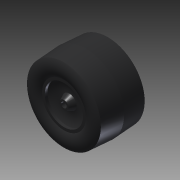
# Autodesk Inventor part: launcher_wheel
Saved by Autodesk Inventor 2013 (Build 170138000, 138)
## iProperties
Created: 2013-07-24
Part Number: launcher_wheel
Material: Generic
Document SubType Name: Modeling
Designer: dkboone
Density: 1 g/cm^3
Author: dkboone
Autodesk Inventor part; units mm, degrees
ref_plane "YZ Plane" through (0, 0, 0) normal (1, 0, 0) x (0, 1, 0)
ref_plane "XZ Plane" through (0, 0, 0) normal (0, 1, 0) x (-1, 0, 0)
ref_plane "XY Plane" through (0, 0, 0) normal (0, 0, 1) x (1, 0, 0)
sketch "Sketch1" plane through (0, 0, 0) normal (1, 0, 0) x (0, 1, 0)
  line L0 (1.5875, -19.05) -> (1.5875, 12.7)
  line L1 (1.5875, 12.7) -> (2.5875, 12.7)
  line L2 (2.5875, 12.7) -> (4.175, 9.525)
  arc A0 (4.175, 9.525) -> (11.1125, 11.1125) centre (5.6612, 18.9827) ccw
  line L3 (11.1125, 11.1125) -> (11.1125, 12.7)
  line L4 (11.1125, 12.7) -> (12.7, 12.7)
  line L5 (21.4312, 12.7) -> (22.225, 0)
  line L6 (18.2563, -12.7) -> (18.2562, 6.35)
  line L7 (18.2562, 6.35) -> (3.9688, 6.35)
  line L8 (3.9688, 6.35) -> (3.9688, -19.05)
  line L9 (3.9688, -19.05) -> (1.5875, -19.05)
  arc A1 (21.4312, 12.7) -> (12.7, 12.7) centre (17.0656, 7.236) ccw
  line L10 (22.225, 0) -> (21.4312, -12.7)
  line L11 (21.4312, -12.7) -> (18.2563, -12.7)
  line L12 (0, -26.6565) -> (0, 26.5892) projected
  point P0 (0, 0)
  dimension "d0" = 1.5875
  dimension "d1" = 1
  dimension "d2" = 3.175
  dimension "d3" = 1.5875
  dimension "d4" = 11.1125
  dimension "d5" = 12.7
  dimension "d6" = 1.5875
  dimension "d7" = 21.4312
  dimension "d8" = 22.225
  dimension "d9" = 12.7
  dimension "d10" = 12.7
  dimension "d11" = 0
  dimension "d13" = 12.7
  dimension "d14" = 21.4312
  dimension "d15" = 3.175
  dimension "d16" = 19.05
  dimension "d17" = 2.3813
  dimension "d18" = 6.35
  dimension "d19" = 6.35
  dimension "d20" = 12.7
  dimension "d21" = 9.5738
  dimension "d22" = 6.9938
  constraints: 24 end point, 4 perpendicular, 4 point on circle, 2 centre point, 2 parallel, 1 vertical
  measures "d0" distance from line of L0 point (0, 0)
  measures "d1" distance of L0.end L1.end
  measures "d2" vertical distance of L2.end L1.end
  measures "d3" horizontal distance of L1.end L2.end
  measures "d4" horizontal distance of L3.end point (0, 0)
  measures "d5" horizontal distance of L4.end point (0, 0)
  measures "d6" distance of L3.start L3.end
  measures "d7" horizontal distance of L5.start point (0, 0)
  measures "d8" distance of L5.end point (0, 0)
  measures "d9" vertical distance of L5.end L5.start
  measures "d10" distance from line of L5.end L4
  measures "d11" vertical distance of point (0, 0) L5.end
  measures "d13" vertical distance of L10.end L5.end
  measures "d14" horizontal distance of point (0, 0) L10.end
  measures "d15" distance of L10.end L6.start
  measures "d16" distance from line of L9 point (0, 0)
  measures "d17" distance between parallel lines of L0 L8
  measures "d18" distance from line of point (0, 0) L7
  measures "d19" vertical distance of L6.end point (0, 0)
  measures "d20" vertical distance of point (0, 0) L0.end
  measures "d21" radius of A0
  measures "d22" radius of A1
revolve "Revolution1" add sketch "Sketch1" angle 360 about axis through (0, 0, -10) along (0, 0, 1)
equation "\"d14\" = d7"
equation "\"d19\" = d18"
body "Solid1"
